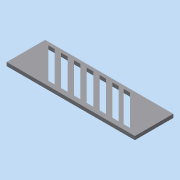
# Autodesk Inventor part: resorte
Saved by Autodesk Inventor 2015 (Build 190159000, 159)
## iProperties
Created: 2017-10-03
Part Number: resorte
Material: Generic
Document SubType Name: Modeling
Designer: macbook
Density: 1 g/cm^3
Appearance: Default
Author: macbook
Autodesk Inventor part; units mm, degrees
ref_plane "YZ Plane" through (0, 0, 0) normal (1, 0, 0) x (0, 1, 0)
ref_plane "XZ Plane" through (0, 0, 0) normal (0, 1, 0) x (-1, 0, 0)
ref_plane "XY Plane" through (0, 0, 0) normal (0, 0, 1) x (1, 0, 0)
sketch "Sketch1" plane through (0, 0, 0) normal (0, 0, 1) x (1, 0, 0)
  line L0 (0, 0) -> (200, 0)
  line L1 (200, 0) -> (200, 60)
  line L2 (200, 60) -> (0, 60)
  line L3 (0, 60) -> (0, 0)
  line L4 (57.7241, 7.2758) -> (67.7241, 7.2758)
  line L5 (67.7241, 7.2758) -> (20.0079, 54.9764)
  line L6 (20.0079, 54.9764) -> (10.0052, 54.979)
  line L7 (10.0052, 54.979) -> (57.7241, 7.2758)
  line L8 (77.7241, 7.2759) -> (87.7451, 7.2759)
  line L9 (87.7451, 7.2759) -> (40.0341, 54.9711)
  line L10 (40.0341, 54.9711) -> (30.0105, 54.9738)
  line L11 (30.0105, 54.9738) -> (77.7241, 7.2759)
  line L12 (50, 54.9738) -> (97.6979, 7.2759)
  line L13 (50, 54.9738) -> (117.455, 54.9738) construction
  line L14 (97.6979, 7.2759) -> (107.6979, 7.2759)
  line L15 (107.6979, 7.2759) -> (60, 54.9738)
  line L16 (107.6979, 7.2759) -> (175.1529, 7.2759) construction
  line L17 (60, 54.9738) -> (50, 54.9738)
  line L18 (70, 54.9738) -> (137.455, 54.9738) construction
  line L19 (90, 54.9738) -> (137.6979, 7.2759)
  line L20 (137.6979, 7.2759) -> (147.6979, 7.2759)
  line L21 (147.6979, 7.2759) -> (100, 54.9738)
  line L22 (100, 54.9738) -> (90, 54.9738)
  line L23 (110, 54.9738) -> (157.6979, 7.2759)
  line L24 (110, 54.9738) -> (177.455, 54.9738) construction
  line L25 (157.6979, 7.2759) -> (167.6979, 7.2759)
  line L26 (167.6979, 7.2759) -> (120, 54.9738)
  line L27 (110, 54.9738) -> (120, 54.9738)
  line L28 (127.455, 54.9738) -> (175.1529, 7.2759)
  line L29 (175.1529, 7.2759) -> (185.1529, 7.2759)
  line L30 (185.1529, 7.2759) -> (137.455, 54.9738)
  line L31 (127.455, 54.9738) -> (137.455, 54.9738)
  line L32 (70, 54.9738) -> (117.6979, 7.2759)
  line L33 (70, 54.9738) -> (137.455, 54.9738) construction
  line L34 (117.6979, 7.2759) -> (127.6979, 7.2759)
  line L35 (127.6979, 7.2759) -> (80, 54.9738)
  line L36 (70, 54.9738) -> (80, 54.9738)
  dimension "d0" = 200
  dimension "d1" = 60
  dimension "d5" = 10
  dimension "d6" = 45
  dimension "d7" = 10
  dimension "d8" = 135
  dimension "d12" = 10
  dimension "d13" = 45
  dimension "d14" = 45
  dimension "d15" = 10
  dimension "d16" = 10
  dimension "d17" = 45
  dimension "d18" = 10
  constraints: 74 end point, 14 point on line, 12 parallel, 10 horizontal, 4 equal length, 2 collinear, 1 perpendicular
  measures "d0" distance of L2.end L1.end
  measures "d1" distance of L0.end L1.end
  measures "d5" distance of L8.start L4.end
  measures "d6" angle of L12 L13
  measures "d7" distance of L12.end L14.end
  measures "d8" angle of L16 L15
  measures "d12" distance of L19.end L20.end
  measures "d13" angle of L21 L20
  measures "d14" angle of L23 L24
  measures "d15" distance of L23.end L25.end
  measures "d16" distance of L16.end L29.end
  measures "d17" angle of L32 L33
  measures "d18" distance of L32.end L34.end
extrude "Extrusion1" add sketch "Sketch1" along normal blind 5.5
body "Solid1"
